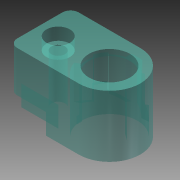
# Autodesk Inventor part: Carcasa (parte 1)
Saved by Autodesk Inventor 2014 (Build 180170000, 170)
## iProperties
Created: 2017-02-07
Part Number: Carcasa (parte 1)
Material: Generic
Document SubType Name: Modeling
Designer: Rubén
Density: 1 g/cm^3
Appearance: Indoor Pool
Author: Rubén
Autodesk Inventor part; units mm, degrees
ref_plane "YZ Plane" through (0, 0, 0) normal (1, 0, 0) x (0, 1, 0)
ref_plane "XZ Plane" through (0, 0, 0) normal (0, 1, 0) x (-1, 0, 0)
ref_plane "XY Plane" through (0, 0, 0) normal (0, 0, 1) x (1, 0, 0)
sketch "Sketch1" plane through (0, 0, 0) normal (0, 1, 0) x (-1, 0, 0)
  circle A0 centre (0, 0) radius 5
  circle A1 centre (0, 0) radius 7.5
  line L0 (0, 7.5) -> (8, 7.5)
  line L1 (17, 4.5) -> (17, -4.5)
  line L2 (8, -7.5) -> (0, -7.5)
  circle A2 centre (12.5, 0) radius 1.65
  line L3 (0, 0) -> (17, 0) construction
  line L4 (17, 4.5) -> (8, 4.5)
  line L5 (8, 4.5) -> (8, 7.5)
  line L6 (17, -4.5) -> (8, -4.5)
  line L7 (8, -4.5) -> (8, -7.5)
  line L8 (8, 4.5) -> (8, -4.5) construction
  line L9 (12.5, 4.5) -> (12.5, -4.5) construction
  dimension "d12" = 10
  dimension "d13" = 15
  dimension "d14" = 8
  dimension "d15" = 3
  dimension "d16" = 3.3
  constraints: 20 end point, 4 midpoint, 4 perpendicular, 3 centre point, 2 coincident, 2 equal length, 2 horizontal, 2 point on circle, 2 tangent, 1 collinear, 1 parallel, 1 point on line, 1 vertical
  measures "d12" diameter of A0
  measures "d13" diameter of A1
  measures "d14" distance from line of L8 point (0, 0)
  measures "d15" distance of L4.end L0.end
  measures "d16" diameter of A2
extrude "Extrusion1" add sketch "Sketch1" along normal blind 15
sketch "Sketch4" plane through (0, 15, 0) normal (0, 1, 0) x (1, 0, 0)
  circle A0 centre (-12.5, 0) radius 1.65 projected
  circle A1 centre (-12.5, 0) radius 2.85
  dimension "d20" = 5.7
  constraints: 1 centre point, 1 coincident
  measures "d20" diameter of A1
extrude "Extrusion4" cut sketch "Sketch4" against normal blind 3
sketch "Sketch5" plane through (0, 15, 0) normal (0, 1, 0) x (1, 0, 0)
  line L0 (-8, 7.5) -> (-8, 4.5) projected
  line L1 (-8, 4.5) -> (-17, 4.5) projected
  line L2 (-17, 4.5) -> (-17, -4.5) projected
  line L3 (-17, -4.5) -> (-8, -4.5) projected
  line L4 (-8, -4.5) -> (-8, -7.5) projected
  line L5 (-8, -7.5) -> (0, -7.5) projected
  line L6 (-8, 7.5) -> (-17, 7.5)
  line L7 (-17, 7.5) -> (-17, 4.5)
  line L8 (-17, -4.5) -> (-17, -7.5)
  line L9 (-17, -7.5) -> (-8, -7.5)
  constraints: 8 end point, 2 collinear, 1 parallel, 1 perpendicular
extrude "Extrusion5" add sketch "Sketch5" against normal blind 10
fillet "Fillet1" radius 2 2 edges at (-17, 10, -7.5) (-17, 10, 7.5)
sketch "Sketch2" plane through (0, 0, 0) normal (0, -1, 0) x (1, 0, 0)
  circle A0 centre (0, 0) radius 5 projected
  arc A1 (0, -7.5) -> (0, 7.5) centre (0, 0) ccw projected
  circle A2 centre (0, 0) radius 5.5
  dimension "d35" = 11
  constraints: 1 centre point, 1 coincident
  measures "d35" diameter of A2
extrude "Extrusion2" cut sketch "Sketch2" against normal blind 13.5
sketch "Sketch6" plane through (0, 0, 0) normal (0, -1, 0) x (1, 0, 0)
  circle A0 centre (0, 0) radius 5.5 projected
  line L0 (0, -7.5) -> (-8, -7.5) projected
  arc A1 (0, -7.5) -> (0, 7.5) centre (0, 0) ccw projected
  line L1 (0, 0) -> (0, 6.8) construction
  arc A2 (1.35, 6.6646) -> (-1.35, 6.6646) centre (0, 0) ccw
  line L2 (-1.35, 6.6646) -> (-1.35, 5.3317)
  line L3 (1.35, 6.6646) -> (1.35, 5.3317)
  arc A3 (1.35, 5.3317) -> (-1.35, 5.3317) centre (0, 0) ccw
  arc A4 (-5.0968, 4.5015) -> (-6.4468, 2.1632) centre (0, 0) ccw
  line L4 (-6.4468, 2.1632) -> (-5.2924, 1.4967)
  line L5 (-5.0968, 4.5015) -> (-3.9424, 3.835)
  arc A5 (-3.9424, 3.835) -> (-5.2924, 1.4967) centre (0, 0) ccw
  arc A6 (-6.4468, -2.1632) -> (-5.0968, -4.5015) centre (0, 0) ccw
  line L6 (-5.0968, -4.5015) -> (-3.9424, -3.835)
  line L7 (-6.4468, -2.1632) -> (-5.2924, -1.4967)
  arc A7 (-5.2924, -1.4967) -> (-3.9424, -3.835) centre (0, 0) ccw
  arc A8 (-1.35, -6.6646) -> (1.35, -6.6646) centre (0, 0) ccw
  line L8 (1.35, -6.6646) -> (1.35, -5.3317)
  line L9 (-1.35, -6.6646) -> (-1.35, -5.3317)
  arc A9 (-1.35, -5.3317) -> (1.35, -5.3317) centre (0, 0) ccw
  arc A10 (5.0968, -4.5015) -> (6.4468, -2.1632) centre (0, 0) ccw
  line L10 (6.4468, -2.1632) -> (5.2924, -1.4967)
  line L11 (5.0968, -4.5015) -> (3.9424, -3.835)
  arc A11 (3.9424, -3.835) -> (5.2924, -1.4967) centre (0, 0) ccw
  arc A12 (6.4468, 2.1632) -> (5.0968, 4.5015) centre (0, 0) ccw
  line L12 (5.0968, 4.5015) -> (3.9424, 3.835)
  line L13 (6.4468, 2.1632) -> (5.2924, 1.4967)
  arc A13 (5.2924, 1.4967) -> (3.9424, 3.835) centre (0, 0) ccw
  point P0 (-5.889, 3.4)
  point P1 (-5.889, -3.4)
  point P2 (0, -6.8)
  point P3 (5.889, -3.4)
  point P4 (5.889, 3.4)
  dimension "d36" = 2.7
  dimension "d37" = 6.8
  dimension "d44" = 360
  constraints: 32 point on circle, 26 end point, 12 centre point, 9 coincident, 3 parallel, 1 perpendicular, 65 other
  measures "d36" distance between parallel lines of L3 L2
  measures "d37" radius of A2
extrude "Extrusion6" cut sketch "Sketch6" against normal up to surface (13.5 mm away) contours A0 L12 A12 L13 | L10 A10 L11 A0 | A0 L2 A2 L3 | L8 A8 L9 A0 | A0 L4 A4 L5 | L6 A6 L7 A0
sketch "Sketch7" plane through (0, 0, 0) normal (0, -1, 0) x (1, 0, 0)
  line L0 (5.2924, -1.4967) -> (6.4468, -2.1632) projected
  arc A0 (5.0968, -4.5015) -> (6.4468, -2.1632) centre (0, 0) ccw projected
  line L1 (5.0968, -4.5015) -> (3.9424, -3.835) projected
  arc A1 (1.35, -5.3317) -> (3.9424, -3.835) centre (0, 0) ccw projected
  line L2 (1.35, -5.3317) -> (1.35, -6.6646) projected
  arc A2 (-1.35, -6.6646) -> (1.35, -6.6646) centre (0, 0) ccw projected
  line L3 (-1.35, -6.6646) -> (-1.35, -5.3317) projected
  arc A3 (-3.9424, -3.835) -> (-1.35, -5.3317) centre (0, 0) ccw projected
  line L4 (-3.9424, -3.835) -> (-5.0968, -4.5015) projected
  arc A4 (-6.4468, -2.1632) -> (-5.0968, -4.5015) centre (0, 0) ccw projected
  line L5 (-6.4468, -2.1632) -> (-5.2924, -1.4967) projected
  arc A5 (-5.2924, 1.4967) -> (-5.2924, -1.4967) centre (0, 0) ccw projected
  line L6 (-5.2924, 1.4967) -> (-6.4468, 2.1632) projected
  arc A6 (-5.0968, 4.5015) -> (-6.4468, 2.1632) centre (0, 0) ccw projected
  line L7 (-5.0968, 4.5015) -> (-3.9424, 3.835) projected
  arc A7 (-1.35, 5.3317) -> (-3.9424, 3.835) centre (0, 0) ccw projected
  line L8 (-1.35, 5.3317) -> (-1.35, 6.6646) projected
  arc A8 (1.35, 6.6646) -> (-1.35, 6.6646) centre (0, 0) ccw projected
  line L9 (1.35, 6.6646) -> (1.35, 5.3317) projected
  arc A9 (3.9424, 3.835) -> (1.35, 5.3317) centre (0, 0) ccw projected
  line L10 (3.9424, 3.835) -> (5.0968, 4.5015) projected
  arc A10 (6.4468, 2.1632) -> (5.0968, 4.5015) centre (0, 0) ccw projected
  line L11 (6.4468, 2.1632) -> (5.2924, 1.4967) projected
  arc A11 (5.2924, -1.4967) -> (5.2924, 1.4967) centre (0, 0) ccw projected
  circle A12 centre (0, 0) radius 6.8
  constraints: 1 coincident, 3 other
extrude "Extrusion7" cut sketch "Sketch7" against normal blind 3.5 contours A11 L11 A12 L0 | A12 L2 A1 L1 | L10 A9 L9 A12 | A12 L4 A3 L3 | L8 A7 L7 A12 | A12 L6 A5 L5
chamfer "Chamfer1" distance 3.7 angle 25 1 edges at (-1.35, 3.5, 5.9982) measured on face at (-1.85, 3.5, 5.9982)
chamfer "Chamfer2" distance 3.7 angle 25 1 edges at (-5.8696, 3.5, 1.83) measured on face at (-6.1196, 3.5, 1.397)
chamfer "Chamfer3" distance 3.7 angle 25 1 edges at (-4.5196, 3.5, -4.1682) measured on face at (-4.2696, 3.5, -4.6012)
chamfer "Chamfer4" distance 3.7 angle 25 1 edges at (1.35, 3.5, -5.9982) measured on face at (1.85, 3.5, -5.9982)
chamfer "Chamfer5" distance 3.7 angle 25 1 edges at (5.8696, 3.5, -1.83) measured on face at (6.1196, 3.5, -1.397)
chamfer "Chamfer6" distance 3.7 angle 25 1 edges at (4.5196, 3.5, 4.1682) measured on face at (4.2696, 3.5, 4.6012)
sketch "Sketch8" plane through (0, 13.5, 0) normal (0, -1, 0) x (1, 0, 0)
  line L0 (1.35, 5.3317) -> (1.35, 6.6646) projected
  arc A0 (1.35, 6.6646) -> (-1.35, 6.6646) centre (0, 0) ccw projected
  line L1 (-1.35, 6.6646) -> (-1.35, 5.3317) projected
  arc A1 (5.0968, -4.5015) -> (6.4468, -2.1632) centre (0, 0) ccw projected
  arc A2 (1.35, 6) -> (-1.35, 6) centre (0, 0) ccw
  arc A3 (1.35, 5.3317) -> (-1.35, 5.3317) centre (0, 0) ccw construction
  line L2 (0, 6.8) -> (0, 6.15) construction
  line L3 (0, 6.15) -> (0, 5.5) construction
  arc A4 (1.35, 6.6646) -> (-1.35, 6.6646) centre (0, 0) ccw
  line L4 (-1.35, 6) -> (-1.35, 6.6646)
  line L5 (1.35, 6) -> (1.35, 6.6646)
  constraints: 9 point on circle, 8 end point, 3 centre point, 3 coincident, 3 collinear, 1 point on line, 1 vertical
extrude "Extrusion8" add sketch "Sketch8" along normal blind 6.5
pattern_circular "Circular Pattern1" count 3 over 360 about axis through (0, 0, 0) along (0, 1, 0) of "Extrusion8"
body "Solid1"
